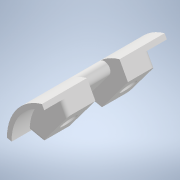
# Autodesk Inventor part: camera fixator
Saved by Autodesk Inventor 2022 (Build 260153000, 153)
## iProperties
Created: 2024-10-14
Part Number: camera fixator
Material: Типовые
Document SubType Name: Modeling
Designer: Andrey
Density: 1 g/cm^3
Appearance: По умолчанию
Author: Andrey
Autodesk Inventor part; units mm, degrees
ref_plane "YZ Plane" through (0, 0, 0) normal (1, 0, 0) x (0, 1, 0)
ref_plane "XZ Plane" through (0, 0, 0) normal (0, 1, 0) x (-1, 0, 0)
ref_plane "XY Plane" through (0, 0, 0) normal (0, 0, 1) x (1, 0, 0)
sketch "Эскиз1" plane through (0, 0, 0) normal (0, 0, 1) x (1, 0, 0)
  arc A0 (-0.8919, 11.7662) -> (-11.5424, -2.4521) centre (0, 0) ccw projected
  line L0 (-0.016, 10.1696) -> (-9.7639, -2.8438) projected
  line L1 (-9.7639, -2.8438) -> (-12.4663, -6.4515) projected
  arc A1 (-0.8919, 11.7662) -> (-11.5424, -2.4521) centre (0, 0) ccw projected
  line L2 (2.8533, 14) -> (-0.016, 10.1696) projected
  arc A2 (-8.5159, 10.4752) -> (-12.3517, -5.4484) centre (0, 0) ccw projected
  circle A3 centre (0, 0) radius 13.5
  circle A4 centre (0, 0) radius 11.8
  circle A5 centre (0, 0) radius 13.3
  circle A6 centre (0, 0) radius 12
  line L3 (-8.1467, 14) -> (2.8533, 14) projected
  line L4 (-8.1467, 14) -> (-8.1467, 11.2511) projected
  arc A7 (-11.5424, -2.4521) -> (-9.7639, -2.8438) centre (-10.5642, -2.2443) ccw projected
  arc A8 (-0.016, 10.1696) -> (-0.8919, 11.7662) centre (-0.8163, 10.7691) ccw projected
  arc A9 (-8.5159, 10.4752) -> (-8.1467, 11.2511) centre (-9.1467, 11.2511) ccw projected
  arc A10 (-12.4663, -6.4515) -> (-12.3517, -5.4484) centre (-13.2667, -5.852) ccw projected
  arc A11 (-11.5424, -2.4521) -> (-9.7639, -2.8438) centre (-10.5642, -2.2443) ccw projected
  arc A12 (-0.016, 10.1696) -> (-0.8919, 11.7662) centre (-0.8163, 10.7691) ccw projected
  point P0 (1.1623, 11.7426)
  point P1 (2.3273, 13.2979)
  point P2 (-11.0819, -4.6034)
  point P3 (1.302, 11.9292)
  point P4 (2.1926, 13.118)
  point P5 (-11.9725, -5.7923)
  dimension "d1" = 0.2
  dimension "d2" = 0.2
  constraints: 2 centre point, 1 coincident, 6 other
extrude "Выдавливание1" add sketch "Эскиз1" along normal mid plane 34 contours A6 L1 A5 L2 picked at (-9.9488, 8.0267)
sketch "Эскиз2" plane through (0, 0, 0) normal (0, 0, 1) x (1, 0, 0)
  arc A0 (-0.8919, 11.7662) -> (-11.5424, -2.4521) centre (0, 0) ccw projected
  line L0 (-0.016, 10.1696) -> (-9.7639, -2.8438) projected
  arc A1 (1.302, 11.9292) -> (-11.0819, -4.6034) centre (0, 0) ccw projected
  line L1 (-14.5944, -9.2926) -> (2.8533, 14) projected
  arc A2 (-11.5424, -2.4521) -> (-9.7639, -2.8438) centre (-10.5642, -2.2443) ccw projected
  arc A3 (-0.016, 10.1696) -> (-0.8919, 11.7662) centre (-0.8163, 10.7691) ccw projected
  point P0 (1.1623, 11.7426)
  point P1 (-10.9422, -4.4168)
extrude "Выдавливание2" add sketch "Эскиз2" along normal mid plane 24
sketch "Эскиз3" plane through (0, 0, 0) normal (0, 0, 1) x (1, 0, 0)
  arc A0 (1.302, 11.9292) -> (-11.0819, -4.6034) centre (0, 0) ccw projected
  line L0 (-11.0819, -4.6034) -> (1.302, 11.9292) projected
  arc A1 (2.1926, 13.118) -> (-11.9725, -5.7923) centre (0, 0) ccw projected
  arc A2 (-8.5159, 10.4752) -> (-12.3517, -5.4484) centre (0, 0) ccw projected
  line L1 (1.302, 11.9292) -> (-11.0819, -4.6034) projected
  line L2 (-4.8899, 3.6629) -> (-10.8048, 8.0935)
  line L3 (-10.8048, 8.0935) -> (-7.6034, 5.6955)
  line L4 (-12.0998, -0.3072) -> (-3.107, 11.6981)
  line L5 (-3.107, 11.6981) -> (0.0944, 9.3001)
  line L6 (0.0944, 9.3001) -> (-8.8984, -2.7053)
  line L7 (-8.8984, -2.7053) -> (-12.0998, -0.3072)
  line L8 (-12.3798, -0.3474) -> (-3.1472, 11.9781)
  line L9 (-3.1472, 11.9781) -> (0.3744, 9.3402)
  line L10 (0.3744, 9.3402) -> (-8.8582, -2.9853)
  line L11 (-8.8582, -2.9853) -> (-12.3798, -0.3474)
  point P0 (-4.402, 3.2974)
  dimension "d7" = 4
  dimension "d8" = 15
  dimension "d9" = 4
  dimension "d12" = 0.2
  dimension "d13" = 15.4
  constraints: 20 end point, 7 perpendicular, 3 midpoint, 2 point on line, 1 point on circle, 3 other
  measures "d7" distance of L3.end L2.end
  measures "d8" distance of L4.start L4.end
  measures "d9" distance of L4.end L5.end
  measures "d12" distance between parallel lines of L7 L11
  measures "d13" distance between parallel lines of L9 L11
extrude "Выдавливание3" cut sketch "Эскиз3" along normal mid plane 9 contours L9 L0 L5 A0 | A0 L5 L4 L8 L9 | L9 L10 L11 L0 L7 L6 L5 | L5 L0 L2 L4 A0 | A0 L4 L5 | L5 L6 L7 L0 | L4 L2 L8 A0 | L0 L7 A0 L4 L2 | L4 A0 L8 L2 | L0 L11 A0 L7 | L4 L7 A0 L11 L8 | A0 L7 L4
sketch "Эскиз5" plane through (0, 0, 17) normal (0, 0, 1) x (1, 0, 0)
  arc A0 (2.1926, 13.118) -> (-11.9725, -5.7923) centre (0, 0) ccw projected
  circle A1 centre (0, 0) radius 13.3
  line L0 (2.8533, 17.048) -> (2.8533, 14) projected
  circle A2 centre (0, 0) radius 2.8533
  line L1 (9.8804, -12.4095) -> (-5.8229, 16.921)
  line L2 (0, 0) -> (2.5154, 1.3467)
  line L3 (-19.8346, 1.2413) -> (17.8745, -6.661)
  line L4 (0, 0) -> (-0.5852, -2.7926)
  line L5 (0, 0) -> (-4.8899, 3.6629)
  line L6 (-0.2736, 9.8256) -> (-9.5063, -2.4999) projected
  point P0 (5.4035, -4.0476)
  point P1 (-13.2994, -0.1282)
  point P2 (-11.9725, -5.7923)
  point P3 (8.6469, -10.1055)
  point P4 (12.1289, -5.457)
  point P5 (-3.6161, 12.799)
  dimension "d19" = 115
  dimension "d20" = 115
  constraints: 10 end point, 2 coincident, 2 point on circle, 2 point on line, 2 tangent, 1 centre point, 1 midpoint, 1 perpendicular, 3 other
  measures "d19" angle of L4 L5
  measures "d20" angle of L2 L5
extrude "Выдавливание5" cut sketch "Эскиз5" against normal blind 40 contours A1 L3 L1 A0 | L3 L1 A1 A0
sketch "Эскиз6" plane through (-8.4854, -1.137, 12) normal (0.8003585, -0.5995217, 0) x (0, 0, -1)
  line L0 (16.5, 0) -> (24, 0) projected
  line L1 (24, 11.9944) -> (24, 0) projected
  line L2 (7.5, 11.9944) -> (0, 11.9944) projected
  line L3 (0, 0) -> (0, 11.9944) projected
  line L4 (16.5, 11.9944) -> (16.5, 0) projected
  line L5 (7.5, 0) -> (7.5, 11.9944) projected
  line L6 (0, 0) -> (0, 11.9944) projected
  line L7 (0, 5.9972) -> (7.5, 5.9972)
  line L8 (7.5, 0) -> (7.5, 11.9944) projected
  line L9 (16.5, 5.9972) -> (24, 5.9972)
  circle A0 centre (3.75, 5.9972) radius 2.1
  circle A1 centre (20.25, 5.9972) radius 2.1
  line L10 (24, 11.9944) -> (16.5, 11.9944) projected
  line L11 (0, 0) -> (7.5, 0) projected
  point P0 (12, 5.9972)
  dimension "d23" = 4.2
  dimension "d24" = 4.2
  constraints: 6 midpoint, 4 end point, 2 centre point, 1 point on line
  measures "d23" diameter of A0
  measures "d24" diameter of A1
extrude "Выдавливание6" cut sketch "Эскиз6" against normal blind 40 contours A1 L9 | L9 A1 | A0 L7 | L7 A0
fillet "Сопряжение2" radius 1 4 edges at (-2.1403, 10.0427, 12) (-10.2393, -0.7695, 12) (-2.1403, 10.0427, -12) (-10.2393, -0.7695, -12)
fillet "Сопряжение3" radius 5 1 edges at (-3.1643, 11.9552, 0)
fillet "Сопряжение4" radius 1.7 1 edges at (-3.6161, 12.799, 0)
